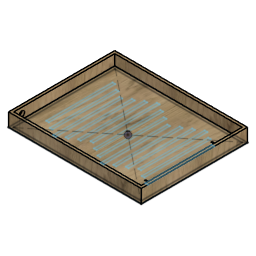
Dissertation_demo v1 (Autodesk Fusion 360 design; units mm, degrees)
Autodesk Fusion 360 part; units mm, degrees
sketch "Sketch1" plane through (0, 0, 0) normal (0, 0, 1) x (1, 0, 0) in component "Component'"
  line L0 (211.4953, 133.158) -> (206.4953, 133.158)
  line L1 (206.4953, 133.158) -> (206.4953, 127.158)
  line L2 (206.4953, 127.158) -> (211.4953, 127.158)
  line L3 (211.4953, 127.158) -> (211.4953, 133.158)
  dimension "d10" = 5
  dimension "d11" = 6
  constraint horizontal L0
  constraint vertical L1
  constraint horizontal L2
  constraint vertical L3
  measures "d10" distance of L0.start L0.end
  measures "d11" distance of L0.start L2.end
extrude "Extrude1" add sketch "Sketch1" against normal blind 3 makes body 1 in component "Component'"
copy_body "CopyPasteBodies1" bodies 1 makes body 2 in component "Component'"
move_body "Move1" bodies 2 to x (1, 0, 0) y (0, 1, 0) z (0, 0, 1) at (0, -17, 0) in component "Component'"
copy_body "CopyPasteBodies2" bodies 1 2 makes body 3 makes body 4 in component "Component'"
move_body "Move2" bodies 3 4 to x (1, 0, 0) y (0, 1, 0) z (0, 0, 1) at (0, -35, 0) in component "Component'"
copy_body "CopyPasteBodies3" bodies 1 2 3 4 makes body 5 makes body 6 makes body 7 makes body 8 in component "Component'"
move_body "Move3" bodies 5 6 7 8 to x (1, 0, 0) y (0, 1, 0) z (0, 0, 1) at (0, -68, 0) in component "Component'"
copy_body "CopyPasteBodies4" bodies 1 2 3 4 5 6 7 makes body 9 makes body 10 makes body 11 makes body 12 makes body 13 makes body 14 makes body 15 in component "Component'"
move_body "Move4" bodies 9 10 11 12 13 14 15 to x (1, 0, 0) y (0, 1, 0) z (0, 0, 1) at (0, -136, 0) in component "Component'"
sketch "Sketch2" plane through (0, 0, 0) normal (0, 0, 1) x (1, 0, 0) in component "Component'"
  line L0 (213.9024, 135.458) -> (203.9024, 135.458)
  line L1 (203.9024, 135.458) -> (203.9024, -114.542)
  line L2 (203.9024, -114.542) -> (213.9024, -114.542)
  line L3 (213.9024, -114.542) -> (213.9024, 135.458)
  dimension "d14" = 10
  dimension "d15" = 250
  constraint horizontal L0
  constraint vertical L1
  constraint horizontal L2
  constraint vertical L3
  measures "d14" distance of L0.start L0.end
  measures "d15" distance of L0.start L2.end
extrude "Extrude2" cut sketch "Sketch2" against normal blind 1 bodies 1 2 3 4 5 6 7 8 9 10 11 12 13 14 15 in component "Component'"
move_body "Move5" bodies 1 2 3 4 5 6 7 9 8 10 12 13 14 15 11 to x (1, 0, 0) y (0, 1, 0) z (0, 0, 1) at (0, 0, -1) in component "Component'"
extrude "Extrude4" add sketch "Sketch2" against normal blind 1 separate body makes body 16 in component "Component'"
sketch "Sketch1 (2)" plane through (0, 0, 0) normal (0, 0, 1) x (1, 0, 0) in component "Main"
  line L0 (-250, 200) -> (250, 200)
  line L1 (250, 200) -> (250, -200)
  line L2 (250, -200) -> (-250, -200)
  line L3 (-250, -200) -> (-250, 200)
  line L4 (-250, 200) -> (250, -200) construction
  line L5 (250, 200) -> (-250, -200) construction
  line L6 (-240, 190) -> (240, 190)
  line L7 (240, 190) -> (240, -190)
  line L8 (240, -190) -> (-240, -190)
  line L9 (-240, -190) -> (-240, 190)
  dimension "d26" = 500
  dimension "d27" = 400
  dimension "d28" = 10
  constraint horizontal L0
  constraint perpendicular L0 L1
  constraint parallel L0 L2
  constraint parallel L1 L3
  constraint coincident L4 origin
  constraint coincident L5 origin
  measures "d26" distance of L1.end L2.end
  measures "d27" distance of L0.end L1.end
extrude "Extrude1'" add sketch "Sketch1 (2)" along normal blind 50 separate body makes body 17 in component "Main"
extrude "Extrude3" add sketch "Sketch1 (2)" along normal blind 10 contours L6 L7 L8 L9 bodies 17 in component "Main"
sketch "Sketch2 (2)" plane through (0, 0, 0) normal (0, 0, 1) x (1, 0, 0) in component "Main"
sketch "Sketch3" plane through (0, 0, 0) normal (0, 0, 1) x (1, 0, 0) in component "Main"
  line L0 (201, 127) -> (189, 127)
  line L1 (189, 127) -> (189, 123)
  line L2 (189, 123) -> (201, 123)
  line L3 (201, 123) -> (201, 127)
  dimension "d35" = 12
  dimension "d36" = 4
  constraint horizontal L0
  constraint vertical L1
  constraint horizontal L2
  constraint vertical L3
  measures "d35" distance of L0.start L0.end
  measures "d36" distance of L0.start L2.end
extrude "Extrude4'" cut sketch "Sketch3" along normal blind 10 bodies 17 in component "Main"
sketch "Sketch4" plane through (-13.9, -10.5, 0) normal (0, 0, 1) x (1, 0, 0) in component "Main"
  line L0 (214.9, -116.5) -> (202.9, -116.5)
  line L1 (202.9, -116.5) -> (202.9, -112.5)
  line L2 (202.9, -112.5) -> (214.9, -112.5)
  line L3 (214.9, -112.5) -> (214.9, -116.5)
  dimension "d39" = 12
  dimension "d40" = 4
  constraint horizontal L0
  constraint vertical L1
  constraint horizontal L2
  constraint vertical L3
  measures "d39" distance of L0.start L0.end
  measures "d40" distance of L0.start L2.end
extrude "Extrude5" cut sketch "Sketch4" along normal blind 10 bodies 17 in component "Main"
sketch "Sketch1 (3)" plane through (0, 0, 0) normal (0, 0, 1) x (1, 0, 0) in component "Component''"
  line L0 (202.6, 125) -> (187.4, 125)
  line L1 (187.4, 125) -> (187.4, -125)
  line L2 (187.4, -125) -> (202.6, -125)
  line L3 (202.6, -125) -> (202.6, 125)
  dimension "d43" = 15.2
  dimension "d44" = 250
  constraint horizontal L0
  constraint vertical L1
  constraint horizontal L2
  constraint vertical L3
  measures "d43" distance of L0.start L0.end
  measures "d44" distance of L0.start L2.end
extrude "Extrude1''" add sketch "Sketch1 (3)" against normal blind 5 separate body makes body 18 in component "Component''"
sketch "Sketch2 (3)" plane through (0, -125, 0) normal (0, -1, 0) x (1, 0, 0) in component "Component''"
  line L0 (202.6, 0) -> (187.4, 0)
  line L1 (187.4, 0) -> (187.4, -5)
  line L2 (187.4, -5) -> (202.6, -5)
  line L3 (202.6, -5) -> (202.6, 0)
  line L4 (202, 0) -> (188, 0)
  line L5 (188, 0) -> (188, -4)
  line L6 (188, -4) -> (202, -4)
  line L7 (202, -4) -> (202, 0)
  constraint horizontal L4
  constraint vertical L5
  constraint horizontal L6
  constraint vertical L7
  constraint coincident L0 L4.start
extrude "Extrude2'" cut sketch "Sketch2 (3)" against normal blind 250 contours L0 L4 L5 L6 L7 bodies 18 in component "Component''"
hole "Hole1" at (-250, -159.5585, 28.611) direction (1, 0, 0) diameter 20 depth 110 tip angle 118 bodies 17 in component "Main"
extrude "Extrude2''" [suppressed] in component "Main"
extrude "Extrude3'" [suppressed] in component "Component'"
sketch "Sketch1 (4)" plane through (0, 0, 0) normal (0, 0, -1) x (1, 0, 0) in component "Component"
  line L0 (140, 190) -> (-140, 190)
  line L1 (-140, 190) -> (-140, -190)
  line L2 (-140, -190) -> (140, -190)
  line L3 (140, -190) -> (140, 190)
  line L4 (120, -150) -> (110, -150)
  line L5 (110, -150) -> (110, 100)
  line L6 (110, 100) -> (120, 100)
  line L7 (120, 100) -> (120, -150)
  dimension "d8" = 10
  dimension "d9" = 250
  constraint horizontal L4
  constraint vertical L5
  constraint horizontal L6
  constraint vertical L7
  measures "d8" distance of L4.start L4.end
  measures "d9" distance of L4.start L6.end
component "Component'" placed x (1, 0, 0) y (0, 1, 0) z (0, 0, 1) at (-13.9, -10.5, 0)
component "Component'" placed x (1, 0, 0) y (0, 1, 0) z (0, 0, 1) at (-43.9, 6.5, 0)
component "Main" placed x (1, 0, 0) y (0, 1, 0) z (0, 0, 1) at (0, 0, 0)
component "Component'" placed x (1, 0, 0) y (0, 1, 0) z (0, 0, 1) at (-73.9, 23.5, 0)
component "Component'" placed x (1, 0, 0) y (0, 1, 0) z (0, 0, 1) at (-103.9, 6.5, 0)
component "Component'" placed x (1, 0, 0) y (0, 1, 0) z (0, 0, 1) at (-133.9, -10.5, 0)
component "Component'" placed x (1, 0, 0) y (0, 1, 0) z (0, 0, 1) at (-163.9, -27.5, 0)
component "Component'" placed x (1, 0, 0) y (0, 1, 0) z (0, 0, 1) at (-193.9, -10.5, 0)
component "Component'" placed x (1, 0, 0) y (0, 1, 0) z (0, 0, 1) at (-223.9, 6.5, 0)
component "Component'" placed x (1, 0, 0) y (0, 1, 0) z (0, 0, 1) at (-253.9, 23.5, 0)
component "Component'" placed x (1, 0, 0) y (0, 1, 0) z (0, 0, 1) at (-283.9, 6.5, 0)
component "Component'" placed x (1, 0, 0) y (0, 1, 0) z (0, 0, 1) at (-313.9, -10.5, 0)
component "Component'" placed x (1, 0, 0) y (0, 1, 0) z (0, 0, 1) at (-343.9, -27.5, 0)
component "Component'" placed x (1, 0, 0) y (0, 1, 0) z (0, 0, 1) at (-373.9, -10.5, 0)
component "Component'" placed x (1, 0, 0) y (0, 1, 0) z (0, 0, 1) at (-403.9, 6.5, 0)
component "Component''" placed x (1, 0, 0) y (0, 1, 0) z (0, 0, 1) at (13.9, 10.5, 0) in component "Component'"
